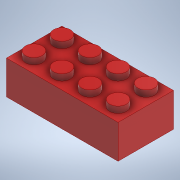
# Autodesk Inventor part: Lego Brick
Saved by Autodesk Inventor 2020 (Build 240168000, 168)
## iProperties
Created: 2021-02-04
Part Number: Lego Brick
Material: Generic
Document SubType Name: Modeling
Designer: Pratishtha  Arya
Density: 1 g/cm^3
Appearance: Red
Author: Pratishtha  Arya
Autodesk Inventor part; units mm, degrees
ref_plane "YZ Plane" through (0, 0, 0) normal (1, 0, 0) x (0, 1, 0)
ref_plane "XZ Plane" through (0, 0, 0) normal (0, 1, 0) x (-1, 0, 0)
ref_plane "XY Plane" through (0, 0, 0) normal (0, 0, 1) x (1, 0, 0)
sketch "Sketch1" plane through (0, 0, 0) normal (0, 1, 0) x (-1, 0, 0)
  line L0 (15.9, 7.9) -> (-15.9, 7.9)
  line L1 (-15.9, 7.9) -> (-15.9, -7.9)
  line L2 (-15.9, -7.9) -> (15.9, -7.9)
  line L3 (15.9, -7.9) -> (15.9, 7.9)
  line L4 (15.9, 7.9) -> (-15.9, -7.9) construction
  line L5 (-15.9, 7.9) -> (15.9, -7.9) construction
  point P0 (0, 0)
  dimension "d0" = 31.8
  dimension "d1" = 15.8
  constraints: 12 end point, 2 midpoint, 2 parallel, 1 horizontal, 1 perpendicular
  measures "d0" distance of L0.start L0.end
  measures "d1" distance of L0.end L1.end
extrude "Extrusion1" add sketch "Sketch1" along normal blind 9.6
sketch "Sketch2" plane through (0, 0, 0) normal (0, -1, 0) x (1, 0, 0)
  line L0 (-14.7, -6.7) -> (14.7, -6.7)
  line L1 (14.7, -6.7) -> (14.7, 6.7)
  line L2 (14.7, 6.7) -> (-14.7, 6.7)
  line L3 (-14.7, 6.7) -> (-14.7, -6.7)
  line L4 (-14.7, -6.7) -> (14.7, 6.7) construction
  line L5 (14.7, -6.7) -> (-14.7, 6.7) construction
  line L6 (-15.9, 7.9) -> (15.9, 7.9) projected
  line L7 (15.9, 7.9) -> (15.9, -7.9) projected
  point P0 (0, 0)
  dimension "d4" = 1.2
  dimension "d5" = 1.2
  constraints: 12 end point, 2 midpoint, 2 parallel, 1 horizontal, 1 perpendicular
  measures "d4" distance between parallel lines of L6 L2
  measures "d5" distance between parallel lines of L7 L1
extrude "Extrusion2" cut sketch "Sketch2" against normal blind 8.6
sketch "Sketch3" plane through (0, 9.6, 0) normal (0, 1, 0) x (1, 0, 0)
  circle A0 centre (12, 4) radius 2.4
  line L0 (15.9, -7.9) -> (15.9, 7.9) projected
  point P0 (0, 0)
  dimension "d8" = 4.8
  dimension "d9" = 3.9
  dimension "d10" = 4
  constraints: 1 centre point
  measures "d8" diameter of A0
  measures "d9" distance from line of L0 A0.centre
  measures "d10" vertical distance of point (0, 0) A0.centre
extrude "Extrusion3" add sketch "Sketch3" along normal blind 1.8
sketch "Sketch4" plane through (0, 8.6, 0) normal (0, -1, 0) x (1, 0, 0)
  circle A0 centre (12, -4) radius 2.4 projected
  point P0 (0, 0)
  constraints: 1 coincident
hole "Hole1" at (12, 8.6, -4) direction (0, 1, 0) diameter 2.6 depth 1.7
pattern_linear "Rectangular Pattern1" count 4 spacing 8 along (-1, 0, 0) count 2 spacing 8 along (0, 0, 1) of "Extrusion3"
pattern_linear "Rectangular Pattern2" count 4 spacing 8 along (-1, 0, 0) count 2 spacing 8 along (0, 0, 1) of "Hole1"
sketch "Sketch5" plane through (0, 8.6, 0) normal (0, -1, 0) x (1, 0, 0)
  circle A0 centre (0, 0) radius 3.255
  circle A1 centre (0, 0) radius 2.4
  dimension "d32" = 6.51
  dimension "d33" = 4.8
  constraints: 2 centre point, 2 coincident
  measures "d32" diameter of A0
  measures "d33" diameter of A1
extrude "Extrusion4" add sketch "Sketch5" along normal up to surface (8.6 mm away)
pattern_linear "Rectangular Pattern3" count 2 spacing 8 along (-1, 0, 0) of "Extrusion4"
pattern_linear "Rectangular Pattern4" count 2 spacing 8 along (1, 0, 0) of "Extrusion4"
sketch "Sketch6" plane through (0, 8.6, 0) normal (0, -1, 0) x (1, 0, 0)
  circle A0 centre (0, 0) radius 3.255 projected
  line L0 (-14.7, 6.7) -> (14.7, 6.7) projected
  line L1 (-0.4, 6.7) -> (-0.4, 3.2303)
  line L2 (0.4, 6.7) -> (0.4, 3.2303)
  dimension "d42" = 0.4
  dimension "d43" = 0.4
  constraints: 4 end point, 2 point on circle, 2 point on line, 2 vertical
  measures "d42" distance from line of point (0, 0) L1
  measures "d43" distance from line of point (0, 0) L2
extrude "Extrusion5" add sketch "Sketch6" along normal blind 6.3 contours A0 L1 L0 L2
mirror "Mirror1" about plane through (0, 0, 0) normal (0, 0, 1) of "Extrusion5"
sketch "Sketch7" plane through (0, 0, 0) normal (0, -1, 0) x (1, 0, 0)
  line L0 (14.7, -6.7) -> (-14.7, -6.7) projected
  line L1 (-12.3, -6.9) -> (-11.7, -6.9)
  line L2 (-11.7, -6.9) -> (-11.7, -6.5)
  line L3 (-11.7, -6.5) -> (-12.3, -6.5)
  line L4 (-12.3, -6.5) -> (-12.3, -6.9)
  line L5 (-12.3, -6.9) -> (-11.7, -6.5) construction
  line L6 (-11.7, -6.9) -> (-12.3, -6.5) construction
  line L7 (-15.9, -7.9) -> (-15.9, 7.9) projected
  point P0 (0, 0)
  point P1 (-12, -6.7)
  dimension "d46" = 3.9
  dimension "d47" = 0.6
  dimension "d48" = 0.4
  constraints: 12 end point, 2 midpoint, 2 parallel, 1 horizontal, 1 perpendicular, 1 point on line
  measures "d46" distance from line of point (-12, -6.7) L7
  measures "d47" distance of L2.end L3.end
  measures "d48" distance of L1.end L2.end
extrude "Extrusion6" add sketch "Sketch7" against normal up to surface (8.6 mm away)
pattern_linear "Rectangular Pattern5" count 4 spacing 8 along (1, 0, 0) of "Extrusion6"
sketch "Sketch8" plane through (0, 8.6, 0) normal (0, -1, 0) x (1, 0, 0)
  line L0 (-14.7, 6.7) -> (14.7, 6.7) projected
  line L1 (12.3, 6.8) -> (11.7, 6.8)
  line L2 (11.7, 6.8) -> (11.7, 6.6)
  line L3 (11.7, 6.6) -> (12.3, 6.6)
  line L4 (12.3, 6.6) -> (12.3, 6.8)
  line L5 (0.4, 6.7) -> (14.7, 6.7) projected
  line L6 (12.3, 6.8) -> (11.7, 6.6) construction
  line L7 (11.7, 6.8) -> (12.3, 6.6) construction
  line L8 (15.9, 7.9) -> (15.9, -7.9) projected
  point P0 (0, 0)
  point P1 (12, 6.7)
  dimension "d54" = 3.9
  dimension "d55" = 0.6
  dimension "d56" = 0.2
  constraints: 12 end point, 2 midpoint, 2 parallel, 1 horizontal, 1 perpendicular, 1 point on line
  measures "d54" distance from line of point (12, 6.7) L8
  measures "d55" distance of L2.end L3.end
  measures "d56" distance of L1.end L2.end
extrude "Extrusion7" add sketch "Sketch8" along normal up to surface (8.6 mm away)
pattern_linear "Rectangular Pattern6" count 4 spacing 8 along (-1, 0, 0) of "Extrusion7"
sketch "Sketch9" plane through (0, 8.6, 0) normal (0, -1, 0) x (1, 0, 0)
  line L0 (-14.5, -3.7) -> (-14.9, -3.7)
  line L1 (-14.9, -3.7) -> (-14.9, -4.3)
  line L2 (-14.9, -4.3) -> (-14.5, -4.3)
  line L3 (-14.5, -4.3) -> (-14.5, -3.7)
  line L4 (-14.7, -6.7) -> (-14.7, 6.7) projected
  line L5 (-14.5, -3.7) -> (-14.9, -4.3) construction
  line L6 (-14.9, -3.7) -> (-14.5, -4.3) construction
  point P0 (0, 0)
  point P1 (-14.7, -4)
  dimension "d62" = 0.6
  dimension "d63" = 0.4
  dimension "d64" = 4
  constraints: 12 end point, 2 midpoint, 2 parallel, 1 horizontal, 1 perpendicular, 1 point on line
  measures "d62" distance of L2.end L0.start
  measures "d63" distance of L1.end L2.end
  measures "d64" vertical distance of point (0, 0) point (-14.7, -4)
extrude "Extrusion8" add sketch "Sketch9" along normal up to surface (8.6 mm away)
pattern_linear "Rectangular Pattern7" count 2 spacing 8 along (0, 0, 1) of "Extrusion8"
sketch "Sketch10" plane through (0, 8.6, 0) normal (0, -1, 0) x (1, 0, 0)
  line L0 (14.7, 6.7) -> (14.7, -6.7) projected
  line L1 (14.9, -3.7) -> (14.5, -3.7)
  line L2 (14.5, -3.7) -> (14.5, -4.3)
  line L3 (14.5, -4.3) -> (14.9, -4.3)
  line L4 (14.9, -4.3) -> (14.9, -3.7)
  line L5 (14.7, 6.7) -> (14.7, -6.7) projected
  line L6 (14.9, -3.7) -> (14.5, -4.3) construction
  line L7 (14.5, -3.7) -> (14.9, -4.3) construction
  point P0 (0, 0)
  point P1 (14.7, -4)
  dimension "d70" = 4
  dimension "d71" = 0.6
  dimension "d72" = 0.4
  constraints: 12 end point, 2 midpoint, 2 parallel, 1 horizontal, 1 perpendicular, 1 point on line
  measures "d70" vertical distance of point (0, 0) point (14.7, -4)
  measures "d71" distance of L1.end L2.end
  measures "d72" distance of L1.start L1.end
extrude "Extrusion9" add sketch "Sketch10" along normal up to surface (8.6 mm away)
mirror "Mirror2" about plane through (0, 0, 0) normal (0, 0, 1) of "Extrusion9"
sketch "Sketch11" plane through (0, 0, 0) normal (0, 1, 0) x (-1, 0, 0)
  point P0 (0, 0)
body "Solid1"
